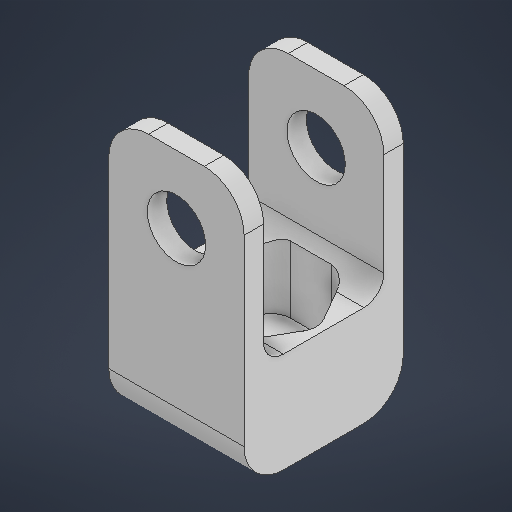
# Autodesk Inventor part: Goal Rush U Joint
Saved by Autodesk Inventor 2025 (Build 290162000, 162)
## iProperties
Created: 2025-02-08
Part Number: Goal Rush U Joint
Material: Generic
Document SubType Name: Modeling
Designer: Juan
Density: 1 g/cm^3
Appearance: Default
Author: Juan
Autodesk Inventor part; units mm, degrees
ref_plane "YZ Plane" through (0, 0, 0) normal (1, 0, 0) x (0, 1, 0)
ref_plane "XZ Plane" through (0, 0, 0) normal (0, 1, 0) x (-1, 0, 0)
ref_plane "XY Plane" through (0, 0, 0) normal (0, 0, 1) x (1, 0, 0)
sketch "Sketch1" plane through (0, 0, 0) normal (0, 1, 0) x (-1, 0, 0)
  circle A0 centre (0, 0) radius 2.3241
  line L0 (0, 0) -> (4.3688, 0)
  line L1 (-5.3975, 6.35) -> (5.3975, 6.35)
  line L2 (5.3975, 6.35) -> (5.3975, -6.35)
  line L3 (5.3975, -6.35) -> (-5.3975, -6.35)
  line L4 (-5.3975, -6.35) -> (-5.3975, 6.35)
  line L5 (-5.3975, 6.35) -> (5.3975, -6.35) construction
  line L6 (5.3975, 6.35) -> (-5.3975, -6.35) construction
  line L7 (0, -6.35) -> (0, -4.7991)
  line L8 (-5.3975, -4.7991) -> (5.3975, -4.7991)
  line L9 (0, 6.35) -> (0, 4.7991)
  line L10 (-5.3975, 4.7991) -> (5.3975, 4.7991)
  line L11 (1.6129, 4.3815) -> (-1.6129, 4.3815)
  line L12 (-1.6129, 4.3815) -> (-1.6129, -4.3815)
  line L13 (-1.6129, -4.3815) -> (1.6129, -4.3815)
  line L14 (1.6129, -4.3815) -> (1.6129, 4.3815)
  line L15 (1.6129, 4.3815) -> (-1.6129, -4.3815) construction
  line L16 (-1.6129, 4.3815) -> (1.6129, -4.3815) construction
  line L17 (2.988, -3.5876) -> (4.6009, -0.7939)
  line L18 (4.6009, 0.7939) -> (2.988, 3.5876)
  line L19 (1.6129, 4.3815) -> (-1.6129, 4.3815)
  line L20 (-2.988, 3.5876) -> (-4.6009, 0.7939)
  line L21 (-4.6009, -0.7939) -> (-2.988, -3.5876)
  arc A1 (-2.988, -3.5876) -> (-1.6129, -4.3815) centre (-1.6129, -2.7936) ccw
  arc A2 (1.6129, -4.3815) -> (2.988, -3.5876) centre (1.6129, -2.7936) ccw
  arc A3 (4.6009, -0.7939) -> (4.6009, 0.7939) centre (3.2258, 0) ccw
  arc A4 (2.988, 3.5876) -> (1.6129, 4.3815) centre (1.6129, 2.7936) ccw
  arc A5 (-1.6129, 4.3815) -> (-2.988, 3.5876) centre (-1.6129, 2.7936) ccw
  arc A6 (-4.6009, 0.7939) -> (-4.6009, -0.7939) centre (-3.2258, 0) ccw
  point P0 (4.6009, -0.7939)
  point P1 (-1.6129, 4.3815)
  dimension "d0" = 4.6482
  dimension "d1" = 4.3688
  dimension "d12" = 12.7
  dimension "d13" = 10.795
  dimension "d20" = 8.763
  dimension "d21" = 3.2258
  dimension "d24" = 360
  dimension "d28" = 360
  constraints: 44 end point, 12 point on circle, 7 centre point, 6 midpoint, 4 parallel, 4 perpendicular, 4 point on line, 3 horizontal, 1 coincident, 1 tangent, 44 other
  measures "d0" diameter of A0
  measures "d1" distance of L0.start L0.end
  measures "d12" distance of L1.end L2.end
  measures "d13" distance of L2.end L3.end
  measures "d20" distance of L11.end L12.end
  measures "d21" distance of L12.end L13.end
extrude "Extrusion4" add sketch "Sketch1" along normal blind 3.175 contours A0 L14 A4 L18 A3 L17 A2 | A0 L12 L11 L14 | L14 L13 L12 A0 | A0 L12 A1 L21 A6 L20 A5 | L1 L9 L10 L4 | L1 L2 L10 L9 | L10 L2 L8 L4 | L8 L7 L3 L4 | L8 L2 L3 L7
extrude "Extrusion5" add sketch "Sketch1" along normal blind 8.001 contours L10 L2 L8 L4
sketch "Sketch3" plane through (0, 3.175, 0) normal (0, 1, 0) x (1, 0, 0)
  line L0 (5.3975, -4.7991) -> (-5.3975, -4.7991) projected
  line L1 (-5.3975, -4.7991) -> (-5.3975, -6.35) projected
  line L2 (-5.3975, -6.35) -> (5.3975, -6.35) projected
  line L3 (5.3975, -6.35) -> (5.3975, -4.7991) projected
  line L4 (-5.3975, 4.7991) -> (5.3975, 4.7991) projected
  line L5 (5.3975, 4.7991) -> (5.3975, 6.35) projected
  line L6 (5.3975, 6.35) -> (-5.3975, 6.35) projected
  line L7 (-5.3975, 6.35) -> (-5.3975, 4.7991) projected
  point P0 (0, 0)
sketch "Sketch4" plane through (-5.3975, 0, 6.35) normal (0, 0, 1) x (1, 0, 0)
  line L0 (0, 0) -> (10.795, 0) projected
  line L1 (10.795, 0) -> (10.795, 3.175) projected
  line L2 (0, 3.175) -> (10.795, 3.175) projected
  line L3 (0, 0) -> (0, 3.175) projected
  line L4 (5.3975, 0) -> (5.3975, 3.175)
  line L5 (5.3975, 1.5875) -> (5.3975, 15.5575)
  circle A0 centre (5.3975, 15.5575) radius 2.3241
  dimension "d34" = 13.97
  dimension "d35" = 4.6482
  constraints: 4 end point, 2 midpoint, 1 centre point, 1 coincident, 1 point on line
  measures "d34" distance of L5.start L5.end
  measures "d35" diameter of A0
extrude "Extrusion6" add sketch "Sketch3" along normal blind 17.78
extrude "Extrusion7" cut sketch "Sketch4" against normal through all contours A0
fillet "Fillet1" radius 3.175 4 edges at (5.3975, 20.955, 5.5745) (-5.3975, 20.955, 5.5745) (5.3975, 20.955, -5.5745) (-5.3975, 20.955, -5.5745)
fillet "Fillet2" radius 1.5875 2 edges at (0, 8.001, 4.7991) (0, 8.001, -4.7991)
fillet "Fillet3" radius 3.175 2 edges at (0, 0, 6.35) (0, 0, -6.35)
body "Solid2"
